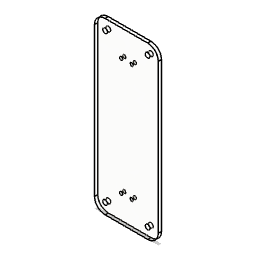
segundo_piso_v6 (Autodesk Fusion 360 design; units mm, degrees)
Autodesk Fusion 360 part; units mm, degrees
sketch "Sketch1" plane through (0, 0, 0) normal (0, 0, 1) x (1, 0, 0)
  line L0 (30, 80) -> (-30, 80)
  line L1 (-30, 80) -> (-30, -80)
  line L2 (-30, -80) -> (30, -80)
  line L3 (30, -80) -> (30, 80)
  line L4 (30, 80) -> (-30, -80) construction
  line L5 (-30, 80) -> (30, -80) construction
  line L6 (20, 70) -> (-20, 70) construction
  line L7 (-20, 70) -> (-20, -70) construction
  line L8 (-20, -70) -> (20, -70) construction
  line L9 (20, -70) -> (20, 70) construction
  line L10 (20, 70) -> (-20, -70) construction
  line L11 (-20, 70) -> (20, -70) construction
  line L12 (0, 0) -> (30, 0) construction
  circle A0 centre (20, 70) radius 2.25
  circle A1 centre (-20, 70) radius 2.25
  circle A2 centre (-20, -70) radius 2.25
  circle A3 centre (20, -70) radius 2.25
  line L13 (-30, 55) -> (30, 55) construction
  line L14 (0, 0) -> (0, 80) construction
  circle A4 centre (5, 55) radius 1.5
  circle A5 centre (-5, 55) radius 1.5
  circle A6 centre (5, -55) radius 1.5
  circle A7 centre (-5, -55) radius 1.5
  dimension "d1" = 160
  dimension "d2" = 60
  dimension "d3" = 40
  dimension "d4" = 140
  dimension "d5" = 4.5
  dimension "d6" = 4.5
  dimension "d11" = 3
  dimension "d12" = 5
  dimension "d13" = 55
  constraint horizontal L0
  constraint perpendicular L0 L1
  constraint parallel L0 L2
  constraint parallel L1 L3
  constraint coincident L4 L12.start
  constraint coincident L5 L12.start
  constraint coincident L12.start L14.start
  constraint horizontal L6
  constraint perpendicular L6 L7
  constraint parallel L6 L8
  constraint parallel L7 L9
  constraint coincident L10 L12.start
  constraint coincident L11 L12.start
  constraint midpoint L3 L12.end
  constraint coincident L6.start L9.end
  constraint coincident L6.end L7.start
  constraint symmetric L12 A0 A3
  constraint symmetric L12 A1 A2
  constraint coincident L1 L13.start
  constraint coincident L3 L13.end
  constraint perpendicular L3 L13
  constraint midpoint L0 L14.end
  constraint coincident L13 A4.centre
  constraint symmetric L14 A4 A5
  constraint symmetric L12 A4 A6
  constraint symmetric L12 A5 A7
  measures "d1" distance of L0.start L2.end
  measures "d2" distance of L1.end L2.end
  measures "d3" distance of L7.end L8.end
  measures "d4" distance of L6.end L7.end
  measures "d5" diameter of A0
  measures "d6" diameter of A1
  measures "d11" diameter of A4
  measures "d12" distance of L14 A4.centre
  measures "d13" distance of L12 L13
extrude "Extrude1" add sketch "Sketch1" against normal blind 3
fillet "Fillet1" radius 10 4 edges at (-30, -80, -1.5) (30, -80, -1.5) (30, 80, -1.5) (-30, 80, -1.5)
equation "d6 = d5"
